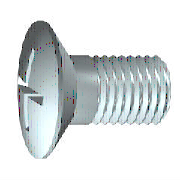
# Autodesk Inventor part: Screw GB/T 820 M3 x 6
Saved by Autodesk Inventor 2015 SP1 (Build 190203100, 203)
## iProperties
Created: 2014-02-16
Part Number: Screw GB/T 820 M3 x 6
Material: Steel, Mild
Description: Cross recessed raised countersunk head screws Type H
Document SubType Name: Modeling
Standard: GB/T 820-2000
Designer: laca
Standard Revision: 2000
Standards Organization: GB
Language: en-US
Size Designation: M3x6
Categories: <MemberInstance><Categories><Category DisplayName="Fasteners" InternalName="e4da775c-781d-43d5-af7c-5136215cf5a6" Mnemonic="FSTN"><Category DisplayName="Bolts" InternalName="536e6df0-f778-49ac-b2f2-25c71d2aa0b2" Mnemonic="SCRW"><CategoryParameter DisplayName="Nominal Diameter Designation" InternalName="03caf894-eafd-4c09-a035-916ac084b87b" Mnemonic="nomdiadesig"/><CategoryParameter DisplayName="Nominal Length" InternalName="238ecbaf-3e6c-45dd-aa95-4068c8e0fd02" Mnemonic="nomlen"/><CategoryParameter DisplayName="Thread Designation" InternalName="586d5e89-370a-4089-914f-0110033585c7" Mnemonic="thrdesign"/><CategoryParameter DisplayName="Thread Series Designation" InternalName="87c5849c-b3a5-4c3e-9c9b-2feecef9be86" Mnemonic="thrserdsgn"/><CategoryParameter DisplayName="Nominal Diameter" InternalName="8bbe3f8e-44cf-40a9-a251-3a6edc8168d6" Mnemonic="nomdia"/><CategoryParameter DisplayName="Thread Type" InternalName="b4bbb7bc-d6aa-4c9f-a9a9-4152b9f6fe49" Mnemonic="thrtype"/><CategoryParameter DisplayName="Thread Pitch" InternalName="bb82302e-82d8-4176-8fc1-c5d7bb17d5ad" Mnemonic="pitch1"/><CategoryParameter DisplayName="Threads per Unit" InternalName="bdc6e7d2-ffd0-4d9c-a173-16b95ebb912d" Mnemonic="thrperunit1"/><CategoryParameter DisplayName="Thread Class" InternalName="ebc0d23b-2cc6-4d2a-b376-d52aae53bab6" Mnemonic="thrclss"/><Category DisplayName="Countersunk" InternalName="49656530-5684-4604-a233-68d537625f23" Mnemonic="CSSCRW"><CategoryParameter DisplayName="Type" InternalName="161b33bb-bee3-4fab-a17d-97511dff40f0" Mnemonic="type"/><CategoryParameter DisplayName="Thread Length" InternalName="207f0278-6dec-43ab-bffc-1c6d03e64de4" Mnemonic="thrlen"/><CategoryParameter DisplayName="Grip Length" InternalName="2fff3de5-ce2a-45fd-9425-99ddc9dff352" Mnemonic="grplen"/><CategoryParameter DisplayName="Property Class" InternalName="5249b721-5ecc-4781-a2e8-d7e3bda3ecca" Mnemonic="propclss"/><CategoryParameter DisplayName="Head Height" InternalName="57526df9-da71-45fb-acb4-1d0529a34778" Mnemonic="headh"/><CategoryParameter DisplayName="Shank Diameter" InternalName="7ece923f-d8ee-40d5-83f8-980cad520964" Mnemonic="grpdia"/><CategoryParameter DisplayName="Head Diameter" InternalName="a509cd31-06d1-44c5-b54e-d7a695352906" Mnemonic="headdia"/><CategoryParameter DisplayName="Head Angle" InternalName="dbcfc1e0-7990-403e-bc2e-90d1c639222a" Mnemonic="headang"/></Category></Category></Category><Category DisplayName="DataType" InternalName="23b78d0f-2648-40c6-8793-ca6db495c9e8" Mnemonic="DATATYPE"><CategoryParameter DisplayName="DisplayName" InternalName="05415f3d-3907-474b-a020-eb9d644f4cf3" Mnemonic="DISPLAYNAME"/><CategoryParameter DisplayName="Standard" InternalName="0c0a119c-1e12-4c84-803f-101930972f5e" Mnemonic="STANDARD"/><CategoryParameter DisplayName="Description" InternalName="13903e3d-64b1-4950-80da-f627842ea37f" Mnemonic="DESCRIPTION"/><CategoryParameter DisplayName="Designation" InternalName="2675968c-4ce5-49e0-a4f5-552d29089031" Mnemonic="DESIGNATION"/><CategoryParameter DisplayName="Default Row" InternalName="2af9ec52-faaa-4026-b378-f9fa4afca842" Mnemonic="DEFAULTROW"/><CategoryParameter DisplayName="Folder Name" InternalName="3f06958e-8713-4116-9be7-ed6184ecc97b" Mnemonic="FOLDERNAME"/><CategoryParameter DisplayName="Revision Guid" InternalName="45a75005-10b1-4dfc-8d6d-dfe629f0b93c" Mnemonic="REVISIONGUID"/><CategoryParameter DisplayName="FileName" InternalName="8b46a4cc-9585-4fed-90c3-899f57e09a73" Mnemonic="FILENAME"/><CategoryParameter DisplayName="StdsOrg" InternalName="8f5914e1-4693-403f-8ab5-d37768198c9d" Mnemonic="STDSORG"/><CategoryParameter DisplayName="Family Version" InternalName="914462f6-6e19-4b14-ba84-155b9680b1d0" Mnemonic="FAMILYREVISION"/><CategoryParameter DisplayName="Standard Revision" InternalName="91d5a463-65c2-4fde-b823-3b7fea5e8e17" Mnemonic="STANDARDREVISION"/><CategoryParameter DisplayName="Member Revision" InternalName="a65d44b9-392f-4f4f-857b-e4b3d54996fe" Mnemonic="MEMBERREVISION"/><CategoryParameter DisplayName="ClipFormat" InternalName="bc51e27b-3422-4e78-93ef-cec197ddf230" Mnemonic="CLIPFORMAT"/><CategoryParameter DisplayName="Manufacturer" InternalName="cd6c7a72-a28a-4e50-99a9-2c7f4e13e5ad" Mnemonic="MANUFACTURER"/><CategoryParameter DisplayName="InternalName" InternalName="cf1d0246-76d9-4b4a-8305-fa0409afb5c1" Mnemonic="INTERNALNAME"/><CategoryParameter DisplayName="IsMetric" InternalName="e2385c5b-1ea4-4823-96a8-8de651266ec3" Mnemonic="ISMETRIC"/><Category DisplayName="Part" InternalName="c0e0b642-3bcb-4cc8-9e80-f96d35c4afa4" Mnemonic="PART"><CategoryParameter DisplayName="Part Number" InternalName="016b6077-bfbe-49bd-92c9-d8d59c39c941" Mnemonic="PARTNUMBER"/><CategoryParameter DisplayName="Stock Number" InternalName="4dba7c1c-e26c-444e-836c-b08b433409a8" Mnemonic="STOCKNUMBER"/><CategoryParameter DisplayName="Material Key" InternalName="5c9a8adb-dd2b-4535-b97f-0a94a95fe41f" Mnemonic="MATERIALKEY"/><CategoryParameter DisplayName="Material" InternalName="818a152a-d3c3-49ca-80ee-df7d91421b8e" Mnemonic="MATERIAL"/></Category></Category><Category DisplayName="LegacyMap" InternalName="cd87c42b-3e48-431e-b5c0-1cbeb14dfe77" Mnemonic="LEGACYMAP"><CategoryParameter DisplayName="unique DA member ID" InternalName="0918ad47-427f-4fed-ae26-24c81c58f590" Mnemonic="DACOOKIE"/><CategoryParameter DisplayName="Merge11 ID" InternalName="0ee8fb18-e2ed-4f39-96f6-1f4b5f50aa71" Mnemonic="MERGE11"/><CategoryParameter DisplayName="unique CC member ID" InternalName="5193edd4-b2b0-4ab4-9d54-de900eee34e0" Mnemonic="CCCOOKIE"/><CategoryParameter DisplayName="Split ID" InternalName="72b5c83c-be7f-45c4-ae51-9160ea6deb26" Mnemonic="SPLIT"/><CategoryParameter DisplayName="MemberID" InternalName="8e5e0294-fc51-4c8f-b3d7-003dc5ed94f6" Mnemonic="MEMBERID"/><CategoryParameter DisplayName="CatalogName" InternalName="d99d1e27-aa94-4de2-af4c-c348882a6f4f" Mnemonic="CATALOGNAME"/><CategoryParameter DisplayName="FamilyNumber" InternalName="e705e1f4-09cb-413e-91f9-551b4188271e" Mnemonic="FAMILYNUMBER"/></Category></Categories><FamilyTemplate Id="si0143"><FamilyTemplateParameters><FamilyTemplateParameter ObjectType="kUserParameterObject" ValueType="xs:double" Id="1" ObjectReferenceKey="GUL"/><FamilyTemplateParameter ObjectType="kUserParameterObject" ValueType="xs:double" Id="2" ObjectReferenceKey="KOH"/><FamilyTemplateParameter ObjectType="kUserParameterObject" ValueType="xs:double" Id="3" ObjectReferenceKey="NLG"/><FamilyTemplateParameter ObjectType="kUserParameterObject" ValueType="xs:double" Id="4" ObjectReferenceKey="KOD"/><FamilyTemplateParameter ObjectType="kUserParameterObject" ValueType="xs:double" Id="5" ObjectReferenceKey="SBR"/><FamilyTemplateParameter ObjectType="kUserParameterObject" ValueType="xs:double" Id="6" ObjectReferenceKey="KR"/><FamilyTemplateParameter ObjectType="kUserParameterObject" ValueType="xs:double" Id="7" ObjectReferenceKey="PTC"/><FamilyTemplateParameter ObjectType="kUserParameterObject" ValueType="xs:double" Id="8" ObjectReferenceKey="GEL"/><FamilyTemplateParameter ObjectType="kUserParameterObject" ValueType="xs:double" Id="9" ObjectReferenceKey="KAH"/><FamilyTemplateParameter ObjectType="kUserParameterObject" ValueType="xs:double" Id="10" ObjectReferenceKey="EPV"/><FamilyTemplateParameter ObjectType="kUserParameterObject" ValueType="xs:double" Id="11" ObjectReferenceKey="THREADDIA"/><FamilyTemplateParameter ObjectType="kUserParameterObject" ValueType="xs:double" Id="12" ObjectReferenceKey="SPD"/><FamilyTemplateParameter ObjectType="kUserParameterObject" ValueType="xs:double" Id="13" ObjectReferenceKey="INTI"/><FamilyTemplateParameter ObjectType="kUserParameterObject" ValueType="xs:double" Id="14" ObjectReferenceKey="BDM"/><FamilyTemplateParameter ObjectType="kUserParameterObject" ValueType="xs:double" Id="15" ObjectReferenceKey="FAWI"/><FamilyTemplateParameter ObjectType="kUserParameterObject" ValueType="xs:double" Id="16" ObjectReferenceKey="RR"/><FamilyTemplateParameter ObjectType="kUserParameterObject" ValueType="xs:double" Id="17" ObjectReferenceKey="TPU"/><FamilyTemplateParameter ObjectType="kUserParameterObject" ValueType="xs:double" Id="18" ObjectReferenceKey="KOHMIN"/><FamilyTemplateParameter ObjectType="kUserParameterObject" ValueType="xs:double" Id="19" ObjectReferenceKey="SDM"/><FamilyTemplateParameter ObjectType="kUserParameterObject" ValueType="xs:double" Id="20" ObjectReferenceKey="NND"/><FamilyTemplateParameter ObjectType="kUserParameterObject" ValueType="xs:double" Id="21" ObjectReferenceKey="GD"/><FamilyTemplateParameter ObjectType="kUserParameterObject" ValueType="xs:double" Id="22" ObjectReferenceKey="SEWI"/><FamilyTemplateParameter ObjectType="kUserParameterObject" ValueType="xs:double" Id="23" ObjectReferenceKey="GAL"/><FamilyTemplateParameter ObjectType="kUserParameterObject" ValueType="xs:double" Id="24" ObjectReferenceKey="TOA"/><FamilyTemplateParameter ObjectType="kUserParameterObject" ValueType="xs:double" Id="25" ObjectReferenceKey="GD1"/><FamilyTemplateParameter ObjectType="kPropertyObject" ValueType="xs:string" Id="100" ObjectReferenceKey="{32853F0F-3444-11d1-9E93-0060B03C1CA6}" SubObjectId="52"/><FamilyTemplateParameter ObjectType="kPropertyObject" ValueType="xs:string" Id="105" ObjectReferenceKey="{32853F0F-3444-11d1-9E93-0060B03C1CA6}" SubObjectId="5"/><FamilyTemplateParameter ObjectType="kPartComponentDefinitionObject" ValueType="xs:string" Id="110" SubObjectId="Material"/><FamilyTemplateParameter ObjectType="kThreadFeatureObject" ValueType="xs:structure" Id="300" ObjectReferenceKey="10020000100000003d0e0000000000008000000000000000" SubObjectId="ThreadInfo"><FamilyTemplateParameter ObjectType="" ValueType="xs:string" Id="301" SubObjectId="ThreadDesignation"/><FamilyTemplateParameter ObjectType="" ValueType="xs:string" Id="302" SubObjectId="ThreadClass"/><FamilyTemplateParameter ObjectType="" ValueType="xs:string" Id="303" SubObjectId="ThreadType"/></FamilyTemplateParameter></FamilyTemplateParameters></FamilyTemplate><CategoryParameterMap><ParamToTemplateMap><ParamToTemplate CategoryParameter="//CategoryParameter[@InternalName='05415f3d-3907-474b-a020-eb9d644f4cf3']" ConstantValue="Screw GB/T 820-2000 Type H"/><ParamToTemplate CategoryParameter="//CategoryParameter[@InternalName='cf1d0246-76d9-4b4a-8305-fa0409afb5c1']" ConstantValue="ec3f025b-3335-4a7d-8323-f831b5f976df"/><ParamToTemplate CategoryParameter="//CategoryParameter[@InternalName='3f06958e-8713-4116-9be7-ed6184ecc97b']" ConstantValue="GB_T 820-2000 H"/><ParamToTemplate CategoryParameter="//CategoryParameter[@InternalName='914462f6-6e19-4b14-ba84-155b9680b1d0']" ConstantValue="10"/><ParamToTemplate CategoryParameter="//CategoryParameter[@InternalName='bc51e27b-3422-4e78-93ef-cec197ddf230']" ConstantValue="CF_INVENTOR.STDPARTS"/><ParamToTemplate CategoryParameter="//CategoryParameter[@InternalName='e2385c5b-1ea4-4823-96a8-8de651266ec3']" ConstantValue="true"/><ParamToTemplate CategoryParameter="//CategoryParameter[@InternalName='13903e3d-64b1-4950-80da-f627842ea37f']" ConstantValue="Cross recessed raised countersunk head screws Type H"/><ParamToTemplate CategoryParameter="//CategoryParameter[@InternalName='8f5914e1-4693-403f-8ab5-d37768198c9d']" ConstantValue="GB"/><ParamToTemplate CategoryParameter="//CategoryParameter[@InternalName='0c0a119c-1e12-4c84-803f-101930972f5e']" ConstantValue="GB/T 820-2000"/><ParamToTemplate CategoryParameter="//CategoryParameter[@InternalName='cd6c7a72-a28a-4e50-99a9-2c7f4e13e5ad']" TemplateParameter="104"/><ParamToTemplate CategoryParameter="//CategoryParameter[@InternalName='91d5a463-65c2-4fde-b823-3b7fea5e8e17']" ConstantValue="2000"/><ParamToTemplate CategoryParameter="//CategoryParameter[@InternalName='45a75005-10b1-4dfc-8d6d-dfe629f0b93c']" ConstantValue="8800f555-daff-45a5-9540-694d7a44aae5"/><ParamToTemplate CategoryParameter="//CategoryParameter[@InternalName='2af9ec52-faaa-4026-b378-f9fa4afca842']" ConstantValue="10"/><ParamToTemplate CategoryParameter="//CategoryParameter[@InternalName='d99d1e27-aa94-4de2-af4c-c348882a6f4f']" ConstantValue="GB"/><ParamToTemplate CategoryParameter="//CategoryParameter[@InternalName='e705e1f4-09cb-413e-91f9-551b4188271e']" ConstantValue="7"/><ParamToTemplate CategoryParameter="//CategoryParameter[@InternalName='8b46a4cc-9585-4fed-90c3-899f57e09a73']" ConstantValue="Screw GB/T 820 M3 x 6"/><ParamToTemplate CategoryParameter="//CategoryParameter[@InternalName='a65d44b9-392f-4f4f-857b-e4b3d54996fe']" ConstantValue="b01627e2-1777-4a5f-83e8-1f600fba6e39"/><ParamToTemplate CategoryParameter="//CategoryParameter[@InternalName='2fff3de5-ce2a-45fd-9425-99ddc9dff352']" ConstantValue="2.7"/><ParamToTemplate CategoryParameter="//CategoryParameter[@InternalName='ebc0d23b-2cc6-4d2a-b376-d52aae53bab6']" ConstantValue="6g"/><ParamToTemplate CategoryParameter="//CategoryParameter[@InternalName='03caf894-eafd-4c09-a035-916ac084b87b']" ConstantValue="M3"/><ParamToTemplate CategoryParameter="//CategoryParameter[@InternalName='b4bbb7bc-d6aa-4c9f-a9a9-4152b9f6fe49']" ConstantValue="GB Metric profile"/><ParamToTemplate CategoryParameter="//CategoryParameter[@InternalName='8e5e0294-fc51-4c8f-b3d7-003dc5ed94f6']" ConstantValue="350"/><ParamToTemplate CategoryParameter="//CategoryParameter[@InternalName='7ece923f-d8ee-40d5-83f8-980cad520964']" TemplateParameter="14"/><ParamToTemplate CategoryParameter="//CategoryParameter[@InternalName='2675968c-4ce5-49e0-a4f5-552d29089031']" TemplateParameter="100"/><ParamToTemplate CategoryParameter="//CategoryParameter[@InternalName='207f0278-6dec-43ab-bffc-1c6d03e64de4']" TemplateParameter="8"/><ParamToTemplate CategoryParameter="//CategoryParameter[@InternalName='a509cd31-06d1-44c5-b54e-d7a695352906']" TemplateParameter="4"/><ParamToTemplate CategoryParameter="//CategoryParameter[@InternalName='57526df9-da71-45fb-acb4-1d0529a34778']" TemplateParameter="2"/><ParamToTemplate CategoryParameter="//CategoryParameter[@InternalName='818a152a-d3c3-49ca-80ee-df7d91421b8e']" TemplateParameter="110"/><ParamToTemplate CategoryParameter="//CategoryParameter[@InternalName='238ecbaf-3e6c-45dd-aa95-4068c8e0fd02']" TemplateParameter="3"/><ParamToTemplate CategoryParameter="//CategoryParameter[@InternalName='8bbe3f8e-44cf-40a9-a251-3a6edc8168d6']" TemplateParameter="20"/><ParamToTemplate CategoryParameter="//CategoryParameter[@InternalName='016b6077-bfbe-49bd-92c9-d8d59c39c941']" TemplateParameter="105"/><ParamToTemplate CategoryParameter="//CategoryParameter[@InternalName='bb82302e-82d8-4176-8fc1-c5d7bb17d5ad']" TemplateParameter="7"/><ParamToTemplate CategoryParameter="//CategoryParameter[@InternalName='dbcfc1e0-7990-403e-bc2e-90d1c639222a']" TemplateParameter="22"/><ParamToTemplate CategoryParameter="//CategoryParameter[@InternalName='586d5e89-370a-4089-914f-0110033585c7']" TemplateParameter="301"/><ParamToTemplate CategoryParameter="//CategoryParameter[@InternalName='bdc6e7d2-ffd0-4d9c-a173-16b95ebb912d']" TemplateParameter="17"/></ParamToTemplateMap></CategoryParameterMap></MemberInstance>
Density: 7.85 g/cm^3
Appearance: Semi-Polished
IsCustomPart: 0
Author: laca
Autodesk Inventor part; units mm, degrees
ref_plane "YZ Plane" through (0, 0, 0) normal (1, 0, 0) x (0, 1, 0)
sketch "Sketch1" plane through (0, 0, 0) normal (0, 0, 1) x (1, 0, 0)
  line L0 (-2.0651, 0) -> (7.3442, 0) projected
  line L1 (0, -1.9685) -> (0, 11.811) projected
  line L2 (6, 0) -> (6, 1.5)
  line L3 (6, 1.5) -> (2.7, 1.5)
  line L4 (-0.1057, 2.75) -> (0, 2.75)
  line L5 (0, 2.75) -> (0, 0) construction
  line L6 (-0.6673, 9.8425) -> (-0.6673, 0) construction
  arc A0 (0, 2.75) -> (-0.4521, 1.5927) centre (5.3327, 0) ccw
  line L7 (-0.4521, 1.5927) -> (0.552, 1.0921)
  line L8 (0.552, 1.0921) -> (1.1327, 0)
  line L9 (1.1327, 0) -> (6, 0)
  line L10 (-0.4521, 1.5927) -> (-0.6673, 1.7) construction
  line L11 (0, 2.75) -> (-0.6673, 2.75)
  line L12 (-0.6673, 0) -> (-0.6673, 2.75)
  arc A1 (-0.4521, 1.5927) -> (-0.6673, 0) centre (5.3327, 0) ccw
  line L13 (0, 2.75) -> (0.2875, 2.75)
  line L14 (0.2875, 2.75) -> (1.7, 1.3375)
  line L15 (1.7, 1.3375) -> (2.3933, 1.3375)
  line L16 (2.3933, 1.3375) -> (2.7, 1.5)
  line L17 (2.7, 1.5) -> (1.5375, 1.5) construction
  dimension "d0" = 6
  dimension "d2" = 0.6673
  dimension "d3" = 3
  dimension "d5" = 1.8
  dimension "d18" = 62
  dimension "d19" = 26.5
  dimension "d20" = 5.5
  dimension "d21" = 3.4
  dimension "d26" = 45
  dimension "d29" = 2.675
  dimension "d30" = 3.3
  dimension "d31" = 0.3067
  dimension "d32" = 1.7
  constraints: 32 end point, 5 collinear, 5 parallel, 4 point on circle, 4 point on line, 3 perpendicular, 2 centre point, 1 coincident, 1 tangent
  measures "d0" distance between parallel lines of L2 L5
  measures "d2" distance between parallel lines of L6 L5
  measures "d3" diameter of L3 L9
  measures "d5" distance from line of L8.end L6
  measures "d18" angle of L8 L9
  measures "d19" angle of L7 L9
  measures "d20" diameter of L4 L9
  measures "d21" diameter of L10.end L9
  measures "d26" angle of L14 L9
  measures "d29" diameter of L15 L9
  measures "d30" distance of L2.end L3.end
  measures "d31" horizontal distance of L15.end L3.end
  measures "d32" distance from line of L14.end L5
revolve "Body" add sketch "Sketch1" angle 360 about axis through (1.1327, 0, 0) along (1, 0, 0) contours L8 L7 L1 L13 L14 L15 L16 L3 L2 L0 | L7 A0 L1
ref_plane "Work Plane1" through (-0.6673, 0, 0) normal (1, 0, 0) x (0, 1, 0)
sketch "Sketch2" plane through (-0.6673, 0, 0) normal (1, 0, 0) x (0, 1, 0)
  circle A0 centre (0, 0) radius 2.75 projected
  line L0 (-4.4845, 0) -> (7.6568, 0) projected
  line L1 (0, -4.4845) -> (0, 7.6568) projected
  line L2 (0, 1.7) -> (0, 0) construction
  line L3 (0, 0) -> (1.7, 0) construction
  line L4 (0, 0) -> (5.9223, 5.9223) construction
  arc A1 (0.51, 0) -> (0, 0.51) centre (0, 0) ccw construction
  arc A2 (1.7, 0) -> (1.6592, 0.37) centre (0, 0) ccw
  arc A3 (0.37, 1.6592) -> (0, 1.7) centre (0, 0) ccw
  arc A4 (1.6592, 0.37) -> (0.37, 1.6592) centre (0, 0) ccw
  arc A5 (1.6592, -0.37) -> (1.7, 0) centre (0, 0) ccw
  arc A6 (0, -1.7) -> (0.37, -1.6592) centre (0, 0) ccw
  arc A7 (0.37, -1.6592) -> (1.6592, -0.37) centre (0, 0) ccw
  arc A8 (-1.6592, 0.37) -> (-1.7, 0) centre (0, 0) ccw
  arc A9 (0, 1.7) -> (-0.37, 1.6592) centre (0, 0) ccw
  arc A10 (-0.37, 1.6592) -> (-1.6592, 0.37) centre (0, 0) ccw
  arc A11 (-0.37, -1.6592) -> (0, -1.7) centre (0, 0) ccw
  arc A12 (-1.6592, -0.37) -> (-0.37, -1.6592) centre (0, 0) ccw
  arc A13 (-1.7, 0) -> (-1.6592, -0.37) centre (0, 0) ccw
  arc A14 (0.5896, 0.0802) -> (0, 0.595) centre (0, 0) ccw construction
  line L5 (1.6592, 0.37) -> (0.5121, 0.303)
  line L6 (0.37, 1.6592) -> (0.303, 0.5121)
  line L7 (0.2767, 0.4284) -> (0.2767, 0.4265)
  arc A15 (0.303, 0.5121) -> (0.5121, 0.303) centre (0.5005, 0.5005) ccw
  arc A16 (1.6592, -0.37) -> (1.7, 0) centre (0, 0) ccw
  arc A17 (0, -1.7) -> (0.37, -1.6592) centre (0, 0) ccw
  arc A18 (0.37, -1.6592) -> (1.6592, -0.37) centre (0, 0) ccw
  line L8 (1.6592, -0.37) -> (0.5121, -0.303)
  line L9 (0.37, -1.6592) -> (0.303, -0.5121)
  arc A19 (0.5121, -0.303) -> (0.303, -0.5121) centre (0.5005, -0.5005) ccw
  arc A20 (-1.6592, 0.37) -> (-1.7, 0) centre (0, 0) ccw
  arc A21 (0, 1.7) -> (-0.37, 1.6592) centre (0, 0) ccw
  arc A22 (-0.37, 1.6592) -> (-1.6592, 0.37) centre (0, 0) ccw
  arc A23 (-0.37, -1.6592) -> (0, -1.7) centre (0, 0) ccw
  arc A24 (-1.6592, -0.37) -> (-0.37, -1.6592) centre (0, 0) ccw
  arc A25 (-1.7, 0) -> (-1.6592, -0.37) centre (0, 0) ccw
  line L10 (-1.6592, 0.37) -> (-0.5121, 0.303)
  line L11 (-0.37, 1.6592) -> (-0.303, 0.5121)
  arc A26 (-0.5121, 0.303) -> (-0.303, 0.5121) centre (-0.5005, 0.5005) ccw
  line L12 (-0.37, -1.6592) -> (-0.303, -0.5121)
  arc A27 (-0.303, -0.5121) -> (-0.5121, -0.303) centre (-0.5005, -0.5005) ccw
  line L13 (-1.6592, -0.37) -> (-0.5121, -0.303)
  dimension "d7" = 45
  dimension "d8" = 1.02
  dimension "d9" = 3.4
  dimension "d10" = 0.37
  dimension "d22" = 1.19
  constraints: 57 point on circle, 27 centre point, 24 end point, 18 symmetric about line, 4 coincident, 3 collinear, 3 point on line, 3 tangent, 1 perpendicular, 27 other
  measures "d7" angle of L4 L3
  measures "d8" diameter of A1
  measures "d9" diameter of A4
  measures "d10" distance from line of L6.start L2
  measures "d22" diameter of A14
extrude "Slot" add sketch "Sketch2" along normal up to next draft 5 contours L5 A15 L6 A4 | A7 L9 A19 L8 | L11 A26 L10 A10 | A12 L13 A27 L12
revolve "Cut" cut sketch "Sketch1" angle 360 about axis through (1.1327, 0, 0) along (1, 0, 0) contours L12 L11 L4 A0 A1
fillet "Fillet1" radius 0.148 5 edges at (-0.4521, 0, 1.5927) (-0.4521, 1.5832, -0.1736) (-0.4521, 1.5832, 0.1736) (-0.4521, 0, -1.5927) (-0.4521, -1.5927, 0)
thread "Thread" size "M3x0.5" designation "M3" class "6g" standard "GB Metric profile" length 3.3
chamfer "Chamfer1" distance 0.3067 distance2 0.3068 1 edges at (6, -1.5, 0) measured on face at (6, -0.4427, -0.5906)
ref_plane "Work Plane3" through (3.0462, 0, 0) normal (0, 1, 0) x (1, 0, 0)
equation "\"d8\" = 0.3 * SDM"
equation "\"d9\" = SDM"
equation "\"d10\" = 0.5 * SBR"
equation "\"d22\" = 0.35 * SDM"
equation "\"d0\" = NLG"
equation "\"d2\" = KAH"
equation "\"d3\" = GD"
equation "\"d5\" = INTI"
equation "\"d20\" = KOD"
equation "\"d21\" = SDM"
equation "\"d26\" = 0.5 * SEWI"
equation "\"d29\" = BDM"
equation "\"d30\" = GEL"
equation "\"d31\" = GAL"
equation "\"d32\" = KOH"
equation "\"d24\" = 0.2 * SBR"
equation "\"d11\" = GEL"
equation "\"d13\" = -0.5 * SPD + 0.5 * GD"
equation "\"GD\" = 3"
equation "\"NLG\" = 6"
equation "\"GEL\" = 3.3"
equation "\"KOD\" = 5.5"
equation "\"KOH\" = 1.7"
equation "\"SDM\" = 3.4"
equation "\"INTI\" = 1.8"
equation "\"SBR\" = 0.74"
equation "\"GUL\" = 0.61345 * PTC"
equation "\"KAH\" = 0.66732"
equation "\"SPD\" = NND - 1.2269 * PTC"
equation "\"SEWI\" = 90deg"
equation "\"d6\" = -KAH"
equation "\"GAL\" = 0.61345 * PTC"
equation "\"BDM\" = 2.675"
equation "\"KR\" = 6"
equation "\"PTC\" = 0.5"
equation "\"EPV\" = 3.2"
equation "\"THREADDIA\" = 3"
equation "\"FAWI\" = 90deg"
equation "\"RR\" = 0.8"
equation "\"KOHMIN\" = 1.25"
equation "\"NND\" = 3"
equation "\"TOA\" = 30deg"
equation "\"GD1\" = THREADDIA - 1.2269 * PTC"
body "Solid1"
